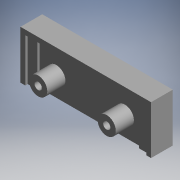
# Autodesk Inventor part: Part2v2
Saved by Autodesk Inventor 2017 (Build 210142000, 142)
## iProperties
Part Number: Part2v2
Material: Generic
Document SubType Name: Modeling
Designer: Ole Simmering
Appearance: Generic
Author: Ole Simmering
Autodesk Inventor part; units mm, degrees
ref_plane "YZ Plane" through (0, 0, 0) normal (1, 0, 0) x (0, 1, 0)
ref_plane "XZ Plane" through (0, 0, 0) normal (0, 1, 0) x (-1, 0, 0)
ref_plane "XY Plane" through (0, 0, 0) normal (0, 0, 1) x (1, 0, 0)
sketch "Sketch1" plane through (0, 0, 0) normal (0, 0, 1) x (1, 0, 0)
  line L0 (0, 0) -> (27, 0)
  line L1 (27, 0) -> (27, 10)
  line L2 (27, 10) -> (0, 10)
  line L3 (0, 10) -> (0, 0)
  dimension "d0" = 27
  dimension "d1" = 10
  constraints: 8 end point, 2 parallel, 1 horizontal, 1 perpendicular
  measures "d0" distance of L2.end L1.end
  measures "d1" distance of L1.end L0.end
extrude "Extrusion1" add sketch "Sketch1" along normal blind 4
sketch "Sketch2" plane through (0, 0, 4) normal (0, 0, 1) x (1, 0, 0)
  line L0 (0, 0) -> (27, 0) projected
  line L1 (0, 0) -> (1, 0)
  line L2 (1, 0) -> (1, 9)
  line L3 (1, 9) -> (26, 9)
  line L4 (26, 9) -> (26, 0)
  line L5 (27, 0) -> (27, 10) projected
  line L6 (27, 0) -> (26, 0)
  line L7 (27, 0) -> (27, 10)
  line L8 (27, 10) -> (0, 10)
  line L9 (0, 10) -> (0, 0) projected
  line L10 (0, 10) -> (0, 0)
  line L11 (13.5, 12) -> (13.5, -6.262) construction
  dimension "d4" = 1
  dimension "d5" = 1
  constraints: 18 end point, 5 perpendicular, 2 point on line, 2 vertical, 1 collinear, 1 other
  measures "d4" distance of L0.start L1.end
  measures "d5" distance between parallel lines of L8 L3
extrude "Extrusion2" add sketch "Sketch2" along normal blind 0.5 contours L9 L8 L5 L0 L4 L3 L2
sketch "Sketch3" plane through (0, 0, 4) normal (0, 0, 1) x (1, 0, 0)
  line L0 (26, 0) -> (26, 9) construction
  line L1 (26, 9) -> (1, 9) construction
  line L2 (1, 9) -> (1, 0) construction
  line L3 (1, 0) -> (26, 0) construction
  line L4 (0, 0) -> (1, 0) construction
  line L5 (1, 0) -> (1, 9) construction
  line L6 (1, 9) -> (26, 9) construction
  line L7 (26, 9) -> (26, 0) construction
  line L8 (26, 0) -> (27, 0) construction
  line L9 (27, 0) -> (27, 10) construction
  line L10 (27, 10) -> (0, 10) construction
  line L11 (0, 10) -> (0, 0) construction
  line L12 (3, 0) -> (24, 0)
  line L13 (0, 0) -> (27, 0) projected
  line L14 (3, 0) -> (3, 9)
  line L15 (24, 0) -> (24, 9)
  line L16 (13.5, 10.7744) -> (13.5, -2.6721) construction
  line L17 (3, 9) -> (24, 9)
  dimension "d8" = 21
  constraints: 10 end point, 3 point on line, 1 horizontal, 1 parallel, 1 perpendicular, 1 vertical, 1 other
  measures "d8" distance of L12.start L12.end
extrude "Extrusion3" cut sketch "Sketch3" against normal blind 0.5
sketch "Sketch4" plane through (0, 0, 3.5) normal (0, 0, 1) x (1, 0, 0)
  line L0 (24, 0) -> (3, 0) construction
  line L1 (24, 9) -> (24, 0) construction
  line L2 (3, 9) -> (24, 9) construction
  line L3 (3, 0) -> (3, 9) construction
  line L4 (3, 0) -> (3, 9) construction
  line L5 (3, 9) -> (1, 9) construction
  line L6 (1, 9) -> (1, 0) construction
  line L7 (1, 0) -> (3, 0) construction
  line L8 (24, 9) -> (24, 0) construction
  line L9 (24, 0) -> (26, 0) construction
  line L10 (26, 0) -> (26, 9) construction
  line L11 (26, 9) -> (24, 9) construction
  line L12 (0, 0) -> (1, 0) construction
  line L13 (1, 0) -> (1, 9) construction
  line L14 (1, 9) -> (26, 9) construction
  line L15 (26, 9) -> (26, 0) construction
  line L16 (26, 0) -> (27, 0) construction
  line L17 (27, 0) -> (27, 10) construction
  line L18 (27, 10) -> (0, 10) construction
  line L19 (0, 10) -> (0, 0) construction
  line L20 (13.5, 12.5235) -> (13.5, -4.7396) construction
  circle A0 centre (6.4125, 4) radius 1.875
  circle A1 centre (20.5875, 4) radius 1.875
  point P0 (13.5, 10.4822)
  dimension "d12" = 4
  dimension "d13" = 14.175
  dimension "d14" = 3.75
  constraints: 2 centre point, 2 end point, 2 symmetric about line, 1 coincident, 1 point on line, 1 vertical, 2 other
  measures "d12" distance from line of L0 point (6.413, 4)
  measures "d13" diameter of point (6.413, 4) L20
  measures "d14" diameter of A0
extrude "Extrusion4" add sketch "Sketch4" along normal blind 3.75
sketch "Sketch5" plane through (6.4125, 4, 7.25) normal (0, 0, 1) x (1, 0, 0)
  circle A0 centre (0, 0) radius 1.875 projected
  circle A1 centre (14.175, 0) radius 1.875 projected
  point P0 (-6.4125, -4)
  constraints: 2 coincident
hole "Hole1" at (6.4125, 4, 7.25) at (20.5875, 4, 7.25) direction (0, 0, -1) diameter 1.5 depth 6 tip angle 118
body "Solid1"
